spessorifrigobosch (Autodesk Fusion 360 design; units mm, degrees)
Autodesk Fusion 360 part; units mm, degrees
sketch "Sketch1" plane through (0, 0, 0) normal (0, 0, 1) x (1, 0, 0)
  line L0 (22.9, -18.5) -> (-22.9, -18.5)
  line L1 (-22.9, -18.5) -> (-22.9, 8.8)
  line L2 (-15.5, 18.5) -> (15.5, 18.5)
  line L3 (22.9, 8.8) -> (22.9, -18.5)
  line L4 (22.9, -18.5) -> (-22.9, 18.5) construction
  line L5 (-22.9, -18.5) -> (22.9, 18.5) construction
  line L6 (0, 18.5) -> (0, -18.5)
  line L7 (10, 14.6) -> (10, 8)
  circle A0 centre (-10, 11.3) radius 3.3
  circle A1 centre (10, 11.3) radius 3.3
  line L8 (-22.9, 8.8) -> (-15.5, 18.5)
  line L9 (22.9, 8.8) -> (15.5, 18.5)
  line L10 (-13.9876, 11.3) -> (-13.3, 11.3)
  line L11 (13.3, 11.3) -> (13.9876, 11.3)
  line L12 (-10, 8.0786) -> (-10, 8)
  dimension "d1" = 45.8
  dimension "d2" = 37
  dimension "d5" = 6.6
  dimension "d6" = 27.3
  constraint horizontal L0
  constraint perpendicular L0 L1
  constraint parallel L0 L2
  constraint parallel L1 L3
  constraint coincident L4 origin
  constraint coincident L5 origin
  constraint midpoint L0 L6.end
  constraint symmetric L6 A0 A1
  constraint symmetric L6 L1.end L3.start
  constraint symmetric L6 L2.start L2.end
  constraint coincident L2 L6.start
  constraint coincident L4 L10.start
  constraint coincident A0 L10.end
  constraint collinear L10 L11
  constraint coincident A1 L11.start
  constraint coincident L5 L11.end
  constraint coincident A0 L12.end
  constraint coincident L4 L12.start
  constraint coincident A1 L7.start
  constraint coincident A1 L7.end
  measures "d1" distance of L4.end L5.end
  measures "d2" distance of L0.end L4.end
  measures "d5" diameter of A0
  measures "d6" distance of L0 L1.end
extrude "Extrude1" add sketch "Sketch1" along normal blind 3
fillet "Fillet1" radius 2.5 6 edges at (15.5, 18.5, 1.5) (22.9, 8.8, 1.5) (22.9, -18.5, 1.5) (-22.9, -18.5, 1.5) (-22.9, 8.8, 1.5) (-15.5, 18.5, 1.5)
